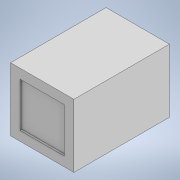
# Autodesk Inventor part: acrylicpmt
Saved by Autodesk Inventor 2022.2 (Build 262287030, 287C)
## iProperties
Created: 2022-02-04
Part Number: acrylicpmt
Material: Generic
Document SubType Name: Modeling
Designer: Tapendra
Density: 1 g/cm^3
Appearance: Default
Author: Tapendra
Autodesk Inventor part; units mm, degrees
ref_plane "YZ Plane" through (0, 0, 0) normal (1, 0, 0) x (0, 1, 0)
ref_plane "XZ Plane" through (0, 0, 0) normal (0, 1, 0) x (-1, 0, 0)
ref_plane "XY Plane" through (0, 0, 0) normal (0, 0, 1) x (1, 0, 0)
sketch "Sketch1" plane through (0, 0, 0) normal (0, 0, 1) x (1, 0, 0)
  line L0 (-16.75, 16.75) -> (16.75, 16.75)
  line L1 (16.75, 16.75) -> (16.75, -16.75)
  line L2 (16.75, -16.75) -> (-16.75, -16.75)
  line L3 (-16.75, -16.75) -> (-16.75, 16.75)
  line L4 (-16.75, 16.75) -> (16.75, -16.75) construction
  line L5 (16.75, 16.75) -> (-16.75, -16.75) construction
  point P0 (0, 0)
  dimension "d0" = 33.5
  dimension "d1" = 33.5
  constraints: 12 end point, 2 midpoint, 2 parallel, 1 horizontal, 1 perpendicular
  measures "d0" distance of L0.start L0.end
  measures "d1" distance of L0.end L1.end
extrude "Extrusion1" add sketch "Sketch1" along normal mid plane 50.5
sketch "Sketch2" plane through (0, 0, 25.25) normal (0, 0, 1) x (1, 0, 0)
  line L0 (-11.75, 11.75) -> (11.75, 11.75)
  line L1 (11.75, 11.75) -> (11.75, -11.75)
  line L2 (11.75, -11.75) -> (-11.75, -11.75)
  line L3 (-11.75, -11.75) -> (-11.75, 11.75)
  line L4 (-11.75, 11.75) -> (11.75, -11.75) construction
  line L5 (11.75, 11.75) -> (-11.75, -11.75) construction
  line L6 (16.75, 16.75) -> (-16.75, 16.75) projected
  line L7 (16.75, -16.75) -> (16.75, 16.75) projected
  point P0 (0, 0)
  dimension "d4" = 5
  dimension "d5" = 5
  constraints: 12 end point, 2 midpoint, 2 parallel, 1 horizontal, 1 perpendicular
  measures "d4" distance between parallel lines of L6 L0
  measures "d5" distance between parallel lines of L7 L1
extrude "Extrusion2" cut sketch "Sketch2" against normal blind 1
sketch "Sketch3" plane through (0, 0, -25.25) normal (0, 0, -1) x (-1, 0, 0)
  point P0 (0, 0)
body "Solid1"
